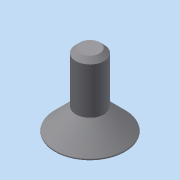
# Autodesk Inventor part: electronicsbox_button
Saved by Autodesk Inventor 2014 (Build 180170000, 170)
## iProperties
Created: 2014-05-26
Part Number: electronicsbox_button
Material: Generic
Document SubType Name: Modeling
Designer: brent
Density: 1 g/cm^3
Appearance: Default
Author: brent
Autodesk Inventor part; units mm, degrees
ref_plane "YZ Plane" through (0, 0, 0) normal (1, 0, 0) x (0, 1, 0)
ref_plane "XZ Plane" through (0, 0, 0) normal (0, 1, 0) x (-1, 0, 0)
ref_plane "XY Plane" through (0, 0, 0) normal (0, 0, 1) x (1, 0, 0)
sketch "Sketch1" plane through (0, 0, 0) normal (0, 1, 0) x (-1, 0, 0)
  circle A0 centre (0, 0) radius 1.6002
  dimension "d0" = 3.2004
  constraints: 1 centre point, 1 coincident
  measures "d0" diameter of A0
extrude "Extrusion1" add sketch "Sketch1" along normal blind 5.715
sketch "Sketch2" plane through (0, 0, 0) normal (0, -1, 0) x (1, 0, 0)
  circle A0 centre (0, 0) radius 1.6002 projected
  circle A1 centre (0, 0) radius 4.1529
  dimension "d3" = 8.3058
  constraints: 1 centre point, 1 coincident
  measures "d3" diameter of A1
extrude "Extrusion2" add sketch "Sketch2" along normal blind 2.54 contours A0 | A1
chamfer "Chamfer1" distance 2.54 angle 45 1 edges at (-4.1529, 0, 0)
fillet "Fillet1" radius 0.127 2 edges at (-4.1529, -2.5399, 0) (-4.1529, -2.54, 0)
chamfer "Chamfer2" distance 0.508 angle 45 1 edges at (1.6002, 5.715, 0)
body "Solid1"
